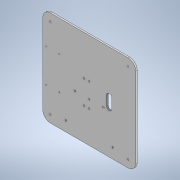
# Autodesk Inventor part: Chassis
Saved by Autodesk Inventor 2020 (Build 240168000, 168)
## iProperties
Created: 2020-02-08
Part Number: Chassis
Material: Generic
Document SubType Name: Modeling
Designer: WIN10
Density: 1 g/cm^3
Appearance: Default
Author: WIN10
Autodesk Inventor part; units mm, degrees
ref_plane "YZ Plane" through (0, 0, 0) normal (1, 0, 0) x (0, 1, 0)
ref_plane "XZ Plane" through (0, 0, 0) normal (0, 1, 0) x (-1, 0, 0)
ref_plane "XY Plane" through (0, 0, 0) normal (0, 0, 1) x (1, 0, 0)
sketch "Sketch1" plane through (0, 0, 0) normal (0, 0, 1) x (1, 0, 0)
  line L0 (-92.5, 40) -> (-92.5, 95)
  line L1 (-92.5, 95) -> (92.5, 95)
  line L2 (92.5, -95) -> (-92.5, -95)
  line L3 (-92.5, -95) -> (-92.5, -40)
  line L4 (-92.5, 95) -> (-62.5, 95)
  line L5 (92.5, 95) -> (62.5, 95)
  line L6 (-92.5, 95) -> (-92.5, 40)
  line L7 (-92.5, -95) -> (-92.5, -40)
  line L8 (92.5, 95) -> (92.5, 40)
  line L9 (92.5, -40) -> (92.5, -95)
  line L10 (-92.5, -95) -> (-77.5, -95)
  line L11 (92.5, -95) -> (77.5, -95)
  line L12 (92.5, 95) -> (77.5, 95)
  line L13 (-92.5, 95) -> (-77.5, 95)
  circle A0 centre (-77.5, 80) radius 1.5
  circle A1 centre (77.5, 80) radius 1.5
  circle A2 centre (-77.5, -80) radius 1.5
  circle A3 centre (77.5, -80) radius 1.5
  circle A4 centre (0, -15) radius 1.5
  line L14 (-92.5, 40) -> (-92.5, -40)
  line L15 (92.5, 40) -> (92.5, -40)
  line L16 (35, 0) -> (35, 15)
  line L17 (35, 15) -> (45, 15)
  line L18 (45, 15) -> (45, -15)
  line L19 (45, -15) -> (35, -15)
  line L20 (35, -15) -> (35, 0)
  line L21 (26.5, -15) -> (26.5, -14)
  line L22 (26.5, -14) -> (29.5, -14)
  line L23 (29.5, -14) -> (29.5, -16)
  line L24 (29.5, -16) -> (26.5, -16)
  line L25 (26.5, -16) -> (26.5, -15)
  line L26 (-26.5, -15) -> (-26.5, -14)
  line L27 (-26.5, -14) -> (-29.5, -14)
  line L28 (-29.5, -14) -> (-29.5, -16)
  line L29 (-29.5, -16) -> (-26.5, -16)
  line L30 (-26.5, -16) -> (-26.5, -15)
  line L31 (-45.5, -75) -> (-45.5, -73.5)
  line L32 (-45.5, -73.5) -> (-47.5, -73.5)
  line L33 (-47.5, -73.5) -> (-47.5, -76.5)
  line L34 (-47.5, -76.5) -> (-45.5, -76.5)
  line L35 (-45.5, -76.5) -> (-45.5, -75)
  line L36 (45.5, -75) -> (45.5, -73.5)
  line L37 (45.5, -73.5) -> (47.5, -73.5)
  line L38 (47.5, -73.5) -> (47.5, -76.5)
  line L39 (47.5, -76.5) -> (45.5, -76.5)
  line L40 (45.5, -76.5) -> (45.5, -75)
  circle A5 centre (-59.5, -33) radius 1
  circle A6 centre (-85.5, -33) radius 1
  circle A7 centre (-85.5, 33) radius 1
  circle A8 centre (-59.5, 33) radius 1
  circle A9 centre (-10, 16) radius 1.5
  circle A10 centre (0, 16) radius 1.5
  circle A11 centre (-10, -31) radius 1.5
  circle A12 centre (0, -31) radius 1.5
  point P0 (0, 0)
  constraints: 82 end point, 23 perpendicular, 13 centre point, 10 point on line, 3 vertical, 2 midpoint, 1 parallel
extrude "Extrusion2" add sketch "Sketch1" along normal blind 3
fillet "Fillet3" radius 15 4 edges at (-92.5, 95, 1.5) (-92.5, -95, 1.5) (92.5, -95, 1.5) (92.5, 95, 1.5)
fillet "Fillet4" radius 5 4 edges at (35, 15, 1.5) (35, -15, 1.5) (45, -15, 1.5) (45, 15, 1.5)
body "Solid2"
